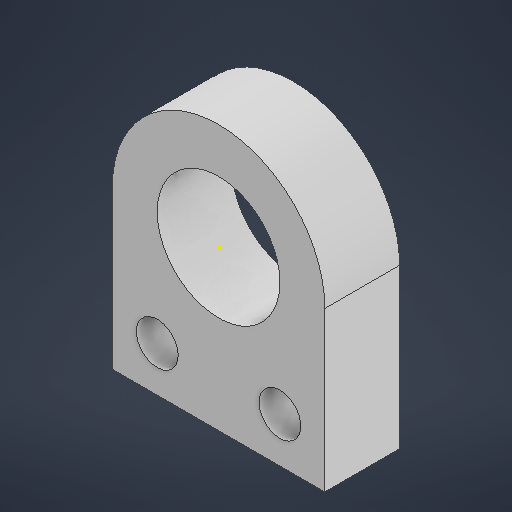
# Autodesk Inventor part: Z轴
Saved by Autodesk Inventor 2025 (Build 290162000, 162)
## iProperties
Created: 2026-04-27
Part Number: Z轴
Material: 常规
Document SubType Name: Modeling
Designer: XH
Density: 1 g/cm^3
Appearance: 默认
Author: XH
Autodesk Inventor part; units mm, degrees
ref_plane "YZ Plane" through (0, 0, 0) normal (1, 0, 0) x (0, 1, 0)
ref_plane "XZ Plane" through (0, 0, 0) normal (0, 1, 0) x (-1, 0, 0)
sketch "草图1" plane through (0, 0, 0) normal (0, 0, 1) x (1, 0, 0)
  circle A0 centre (0, 0) radius 4.1
  circle A1 centre (0, 0) radius 7.1
  dimension "d0" = 8.2
  dimension "d1" = 3
  constraints: 2 centre point, 1 coincident
  measures "d0" diameter of A0
  measures "d1" radial gap between concentric circles of A0 A1
extrude "拉伸1" add sketch "草图1" along normal blind 5
sketch "草图2" plane through (0, 0, 5) normal (0, 0, 1) x (1, 0, 0)
  point P0 (0, 0)
sketch "草图3" plane through (0, 0, 5) normal (0, 0, 1) x (1, 0, 0)
  circle A0 centre (0, 0) radius 7.1 projected
  line L0 (-7.1, 0) -> (7.1, 0)
  line L1 (7.1, 0) -> (7.1, -10.6214)
  line L2 (7.1, -10.6214) -> (-7.1, -10.6214)
  line L3 (-7.1, -10.6214) -> (-7.1, 0)
  line L4 (-7.9158, -10.621) -> (28.0842, -10.6393) projected
  point P0 (7.1, 0)
  constraints: 8 end point, 2 parallel, 1 horizontal, 1 perpendicular, 1 point on line, 2 other
extrude "拉伸2" add sketch "草图3" against normal blind 5 contours L1 L2 L3 A0
sketch "草图4" plane through (0, 0, 5) normal (0, 0, 1) x (1, 0, 0)
  circle A0 centre (-4.1, -7.6214) radius 1.4
  line L0 (-7.1, -10.6214) -> (7.1, -10.6214) projected
  line L1 (-7.1, 0) -> (-7.1, -10.6214) projected
  point P0 (0, 0)
  dimension "d6" = 2.8
  dimension "d7" = 3
  dimension "d8" = 3
  constraints: 1 centre point
  measures "d6" diameter of A0
  measures "d7" distance from line of A0.centre L0
  measures "d8" distance from line of A0.centre L1
extrude "拉伸3" cut sketch "草图4" against normal blind 5
ref_plane "工作平面1" through (0, -10.6214, 5) normal (1, 0, 0) x (0, 0, -1)
mirror "镜像1" about plane through (0, -10.6214, 5) normal (1, 0, 0) of "拉伸3"
